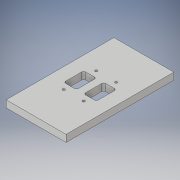
# Autodesk Inventor part: TFPX Plate
Saved by Autodesk Inventor 2019.4 (Build 234330000, 330)
## iProperties
Created: 2020-11-12
Part Number: TFPX Plate
Material: Generic
Document SubType Name: Modeling
Designer: caleb
Density: 1 g/cm^3
Appearance: Default
Author: caleb
Autodesk Inventor part; units mm, degrees
ref_plane "YZ Plane" through (0, 0, 0) normal (1, 0, 0) x (0, 1, 0)
ref_plane "XZ Plane" through (0, 0, 0) normal (0, 1, 0) x (-1, 0, 0)
ref_plane "XY Plane" through (0, 0, 0) normal (0, 0, 1) x (1, 0, 0)
sketch "Sketch5" plane through (0, 0, 0) normal (0, 1, 0) x (-1, 0, 0)
  line L0 (-60, 108) -> (60, 108)
  line L1 (60, 108) -> (60, -108)
  line L2 (60, -108) -> (-60, -108)
  line L3 (-60, -108) -> (-60, 108)
  line L4 (-60, 108) -> (60, -108) construction
  line L5 (60, 108) -> (-60, -108) construction
  point P0 (0, 0)
  dimension "d44" = 216
  dimension "d45" = 120
  constraints: 12 end point, 2 midpoint, 2 parallel, 1 horizontal, 1 perpendicular
  measures "d44" distance of L0.end L1.end
  measures "d45" distance of L1.end L2.end
extrude "Extrusion4" add sketch "Sketch5" along normal blind 14
sketch "Sketch6" plane through (0, 14, 0) normal (0, 1, 0) x (1, 0, 0)
  line L0 (-60, 108) -> (-60, -108) projected
  line L1 (-60, -108) -> (60, -108) projected
  point P0 (0, 0)
  point P1 (-20, -32.5)
  point P2 (-20, 32.5)
  point P3 (20, -32.5)
  point P4 (20, 32.5)
  dimension "d48" = 32.5
  dimension "d51" = 65
  dimension "d54" = 40
  dimension "d57" = 20
  constraints: 1 horizontal, 1 vertical, 3 other
  measures "d48" vertical distance of point (0, 0) point (-20, -32.5)
  measures "d51" distance of point (-20, -32.5) point (-20, 32.5)
  measures "d54" distance of point (-20, -32.5) point (20, -32.5)
  measures "d57" horizontal distance of point (0, 0) point (-20, -32.5)
hole "Hole2" at (-20, 14, 32.5) at (20, 14, 32.5) at (20, 14, -32.5) at (-20, 14, -32.5) direction (0, -1, 0) diameter 4.7625 end through all
sketch "Sketch7" plane through (0, 14, 0) normal (0, 1, 0) x (1, 0, 0)
  line L0 (-11.3, -20) -> (-28.7, -20)
  line L1 (-32.7, -16) -> (-32.7, 16)
  line L2 (-28.7, 20) -> (-11.3, 20)
  line L3 (-7.3, 16) -> (-7.3, -16)
  line L4 (-7.3, -20) -> (-32.7, 20) construction
  line L5 (-32.7, -20) -> (-7.3, 20) construction
  circle A0 centre (-20, -32.5) radius 2.3813 projected
  arc A1 (-32.7, -16) -> (-28.7, -20) centre (-28.7, -16) ccw
  arc A2 (-11.3, -20) -> (-7.3, -16) centre (-11.3, -16) ccw
  arc A3 (-7.3, 16) -> (-11.3, 20) centre (-11.3, 16) ccw
  arc A4 (-28.7, 20) -> (-32.7, 16) centre (-28.7, 16) ccw
  line L6 (-60, -108) -> (60, -108) projected
  arc A5 (28.7, -20) -> (32.7, -16) centre (28.7, -16) ccw
  arc A6 (7.3, -16) -> (11.3, -20) centre (11.3, -16) ccw
  line L7 (28.7, -20) -> (11.3, -20)
  line L8 (7.3, -16) -> (7.3, 16)
  line L9 (32.7, 16) -> (32.7, -16)
  line L10 (32.7, -20) -> (7.3, 20) construction
  line L11 (7.3, -20) -> (32.7, 20) construction
  arc A7 (32.7, 16) -> (28.7, 20) centre (28.7, 16) ccw
  line L12 (11.3, 20) -> (28.7, 20)
  arc A8 (11.3, 20) -> (7.3, 16) centre (11.3, 16) ccw
  point P0 (0, 0)
  point P1 (-20, 0)
  point P2 (-20, 0)
  point P3 (20, 0)
  point P4 (20, 0)
  dimension "d65" = 40
  dimension "d66" = 25.4
  dimension "d67" = 4
  dimension "d70" = 40
  constraints: 24 end point, 16 point on circle, 16 point on line, 8 centre point, 8 tangent, 5 midpoint, 3 equal radius, 2 horizontal, 2 parallel, 1 perpendicular, 1 vertical alignment, 28 other
  measures "d65" distance of L5.start L4.end
  measures "d66" distance of L4.start L5.start
  measures "d67" radius of A1
  measures "d70" distance of A2.centre A5.centre
extrude "Extrusion5" cut sketch "Sketch7" against normal through all contours L0 A1 L1 A4 L2 A3 L3 A2 | L7 A6 L8 A8 L12 A7 L9 A5
sketch "Sketch8" plane through (0, 0, 0) normal (0, -1, 0) x (1, 0, 0)
  line L0 (-46, 98) -> (46, 98)
  line L1 (50, 94) -> (50, -94)
  line L2 (46, -98) -> (-46, -98)
  line L3 (-50, -94) -> (-50, 94)
  line L4 (-50, 98) -> (50, -98) construction
  line L5 (50, 98) -> (-50, -98) construction
  line L6 (60, 108) -> (-60, 108) projected
  line L7 (60, -108) -> (60, 108) projected
  line L8 (7.3, -16) -> (7.3, 16) projected
  line L9 (28.7, -20) -> (11.3, -20) projected
  line L10 (32.7, 16) -> (32.7, -16) projected
  line L11 (11.3, 20) -> (28.7, 20) projected
  arc A0 (50, 94) -> (46, 98) centre (46, 94) ccw
  arc A1 (46, -98) -> (50, -94) centre (46, -94) ccw
  arc A2 (-50, -94) -> (-46, -98) centre (-46, -94) ccw
  arc A3 (-46, 98) -> (-50, 94) centre (-46, 94) ccw
  line L12 (6.5, 37.5) -> (33.5, 37.5)
  line L13 (37.5, 33.5) -> (37.5, -33.5)
  line L14 (33.5, -37.5) -> (6.5, -37.5)
  line L15 (2.5, -33.5) -> (2.5, 33.5)
  line L16 (2.5, 37.5) -> (37.5, -37.5) construction
  line L17 (37.5, 37.5) -> (2.5, -37.5) construction
  arc A4 (37.5, 33.5) -> (33.5, 37.5) centre (33.5, 33.5) ccw
  arc A5 (6.5, 37.5) -> (2.5, 33.5) centre (6.5, 33.5) ccw
  arc A6 (2.5, -33.5) -> (6.5, -37.5) centre (6.5, -33.5) ccw
  arc A7 (33.5, -37.5) -> (37.5, -33.5) centre (33.5, -33.5) ccw
  line L18 (-2.5, 33.5) -> (-2.5, -33.5)
  line L19 (-37.5, -33.5) -> (-37.5, 33.5)
  line L20 (-2.5, 37.5) -> (-37.5, -37.5) construction
  line L21 (-37.5, 37.5) -> (-2.5, -37.5) construction
  line L22 (-90, 98) -> (10, -98) construction
  line L23 (10, 98) -> (-90, -98) construction
  arc A8 (-2.5, 33.5) -> (-6.5, 37.5) centre (-6.5, 33.5) ccw
  arc A9 (-33.5, 37.5) -> (-37.5, 33.5) centre (-33.5, 33.5) ccw
  line L24 (-33.5, 37.5) -> (-6.5, 37.5)
  arc A10 (-37.5, -33.5) -> (-33.5, -37.5) centre (-33.5, -33.5) ccw
  line L25 (-6.5, -37.5) -> (-33.5, -37.5)
  arc A11 (-6.5, -37.5) -> (-2.5, -33.5) centre (-6.5, -33.5) ccw
  point P0 (0, 0)
  point P1 (20, 0)
  point P2 (20, 0)
  point P3 (0, 0)
  point P4 (-11.3, -20)
  point P5 (-32.7, -16)
  point P6 (-20, 0)
  point P7 (-20, 0)
  point P8 (-11.3, 20)
  point P9 (-32.7, 16)
  point P10 (-28.7, 20)
  point P11 (-40, 0)
  point P12 (-40, 0)
  point P13 (-7.3, 16)
  point P14 (-7.3, -16)
  point P15 (-28.7, -20)
  dimension "d77" = 10
  dimension "d78" = 10
  dimension "d79" = 4
  dimension "d80" = 75
  dimension "d81" = 20
  dimension "d82" = 35
  dimension "d83" = 4
  dimension "d86" = 40
  constraints: 40 end point, 24 point on circle, 24 point on line, 16 tangent, 12 centre point, 10 midpoint, 6 equal radius, 4 parallel, 3 horizontal, 2 perpendicular, 1 horizontal alignment, 44 other
  measures "d77" distance between parallel lines of L7 L1
  measures "d78" distance between parallel lines of L6 L0
  measures "d79" radius of A0
  measures "d80" distance of L17.start L16.end
  measures "d81" distance of point (0, 0) point (20, 0)
  measures "d82" distance of L16.end L17.end
  measures "d83" radius of A4
  measures "d86" distance of L9.start point (-11.3, -20)
extrude "Extrusion6" cut sketch "Sketch8" against normal blind 8
body "Solid2"
